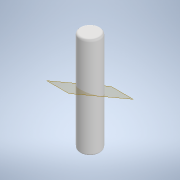
# Autodesk Inventor part: 76. Стопор
Saved by Autodesk Inventor 2021 (Build 250183000, 183)
## iProperties
Created: 2021-04-09
Part Number: 76. Стопор
Material: Типовые
Document SubType Name: Modeling
Designer: Данил
Density: 1 g/cm^3
Appearance: По умолчанию
Author: Данил
Autodesk Inventor part; units mm, degrees
ref_plane "YZ Plane" through (0, 0, 0) normal (1, 0, 0) x (0, 1, 0)
ref_plane "XY Plane" through (0, 0, 0) normal (0, 0, 1) x (1, 0, 0)
sketch "Эскиз1" plane through (0, 0, 0) normal (0, 0, 1) x (1, 0, 0)
  line L0 (0, 12.5) -> (0, -12.5)
  line L1 (0, 12.5) -> (2.5, 12.5)
  line L2 (2.5, 12.5) -> (2.5, -12.5)
  line L3 (2.5, -12.5) -> (0, -12.5)
  line L4 (0, -12.5) -> (0, 12.5)
  point P0 (0, 0)
  point P1 (0, 0)
  dimension "d0" = 25
  dimension "d1" = 5
  constraints: 10 end point, 2 parallel, 1 coincident, 1 horizontal, 1 horizontal alignment, 1 midpoint, 1 perpendicular, 1 vertical
  measures "d0" distance of L0.start L0.end
  measures "d1" diameter of L2 L0
revolve "Вращение1" add sketch "Эскиз1" angle 360 about axis through (0, 12.5, 0) along (0, -1, 0)
fillet "Сопряжение1" radius 0.5 2 edges at (-2.5, 12.5, 0) (-2.5, -12.5, 0)
ref_plane "РабПлоскость1" through (0, 0, 0) normal (0, 0.8660254, -0.5) x (1, 0, 0)
